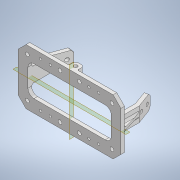
# Autodesk Inventor part: body_shell_1
Saved by Autodesk Inventor 2023 (Build 270158000, 158)
## iProperties
Created: 2021-02-28
Part Number: body_shell_1
Material: Generic
Document SubType Name: Modeling
Designer: Shuang Peng
Density: 1 g/cm^3
Appearance: Default
Author: Shuang Peng
Autodesk Inventor part; units mm, degrees
ref_plane "YZ Plane" through (0, 0, 0) normal (1, 0, 0) x (0, 1, 0)
ref_plane "XZ Plane" through (0, 0, 0) normal (0, 1, 0) x (-1, 0, 0)
ref_plane "XY Plane" through (0, 0, 0) normal (0, 0, 1) x (1, 0, 0)
sketch "Sketch1" plane through (0, 0, 0) normal (0, 0, 1) x (1, 0, 0)
  line L0 (0, -11) -> (-2, -13) projected
  line L1 (0, -4) -> (0, -11) projected
  line L2 (0, 0) -> (0, -4) projected
  line L3 (-15, 0) -> (0, 0) projected
  line L4 (-15, 0) -> (-15, -4) projected
  line L5 (-15, -4) -> (-15, -11) projected
  line L6 (-13, -13) -> (-15, -11) projected
  line L7 (-2, -13) -> (-13, -13) projected
  circle A0 centre (-3.5, -8.5) radius 1.6 projected
  circle A1 centre (-11.5, -8.5) radius 1.6 projected
  line L8 (25, -11) -> (27, -13) projected
  line L9 (27, -13) -> (38, -13) projected
  line L10 (38, -13) -> (40, -11) projected
  line L11 (40, -4) -> (40, -11) projected
  line L12 (40, 0) -> (40, -4) projected
  line L13 (40, 0) -> (25, 0) projected
  line L14 (25, 0) -> (25, -4) projected
  line L15 (25, -4) -> (25, -11) projected
  circle A2 centre (28.5, -8.5) radius 1.6 projected
  circle A3 centre (36.5, -8.5) radius 1.6 projected
  line L16 (0, 31) -> (-2, 33) projected
  line L17 (-2, 33) -> (-13, 33) projected
  line L18 (-13, 33) -> (-15, 31) projected
  line L19 (-15, 24) -> (-15, 31) projected
  line L20 (-15, 20) -> (-15, 24) projected
  line L21 (-15, 20) -> (0, 20) projected
  line L22 (0, 20) -> (0, 24) projected
  line L23 (0, 24) -> (0, 31) projected
  circle A4 centre (-3.5, 28.5) radius 1.6 projected
  circle A5 centre (-11.5, 28.5) radius 1.6 projected
  line L24 (25, 31) -> (27, 33) projected
  line L25 (25, 24) -> (25, 31) projected
  line L26 (25, 20) -> (25, 24) projected
  line L27 (40, 20) -> (25, 20) projected
  line L28 (40, 20) -> (40, 24) projected
  line L29 (40, 24) -> (40, 31) projected
  line L30 (38, 33) -> (40, 31) projected
  line L31 (27, 33) -> (38, 33) projected
  circle A6 centre (28.5, 28.5) radius 1.6 projected
  circle A7 centre (36.5, 28.5) radius 1.6 projected
  line L32 (-11.5, -8.5) -> (-3.5, -8.5)
  line L33 (28.5, -8.5) -> (36.5, -8.5)
  line L34 (-11.5, 28.5) -> (-3.5, 28.5)
  line L35 (28.5, 28.5) -> (36.5, 28.5)
  line L36 (28.5, -8.5) -> (-3.5, -8.5)
  line L37 (-3.5, 28.5) -> (28.5, 28.5)
  line L38 (-15, -14.5) -> (-15, -2.5)
  line L39 (-15, -2.5) -> (40, -2.5)
  line L40 (40, -2.5) -> (40, -14.5)
  line L41 (40, -14.5) -> (-15, -14.5)
  line L42 (-15, -14.5) -> (40, -2.5) construction
  line L43 (-15, -2.5) -> (40, -14.5) construction
  line L44 (-15, 22.5) -> (-15, 34.5)
  line L45 (-15, 34.5) -> (40, 34.5)
  line L46 (40, 34.5) -> (40, 22.5)
  line L47 (40, 22.5) -> (-15, 22.5)
  line L48 (-15, 22.5) -> (40, 34.5) construction
  line L49 (-15, 34.5) -> (40, 22.5) construction
  line L50 (-15, -14.5) -> (-25, -14.5)
  line L51 (-25, -14.5) -> (-25, 34.5)
  line L52 (-25, 34.5) -> (-15, 34.5)
  line L53 (-15, 34.5) -> (-15, -14.5)
  line L54 (40, -14.5) -> (50, -14.5)
  line L55 (50, -14.5) -> (50, 34.5)
  line L56 (50, 34.5) -> (40, 34.5)
  line L57 (40, 34.5) -> (40, -14.5)
  point P0 (12.5, -8.5)
  point P1 (12.5, 28.5)
  point P2 (-15, -2.5)
  dimension "d0" = 12
  dimension "d1" = 55
  dimension "d2" = 12
  dimension "d3" = 55
  dimension "d4" = 10
  dimension "d5" = 49
  dimension "d6" = 10
  dimension "d7" = 49
  constraints: 52 end point, 9 parallel, 7 perpendicular, 6 horizontal, 6 midpoint
  measures "d0" distance of L38.start L38.end
  measures "d1" distance of L38.end L39.end
  measures "d2" distance of L44.start L44.end
  measures "d3" distance of L44.end L45.end
  measures "d4" distance of L51.end L52.end
  measures "d5" distance of L50.end L51.end
  measures "d6" distance of L55.end L56.end
  measures "d7" distance of L54.end L55.end
extrude "Extrusion1" add sketch "Sketch1" along normal blind 3 contours L1 L36 L15 L8 L9 L10 L40 L41 L38 L6 L7 L0 | L0 L7 L6 L5 L4 L39 L2 L1 | L1 L2 L39 L14 L15 L36 | L15 L14 L39 L12 L11 L10 L9 L8 | L38 L50 L51 L52 L44 L19 L20 L53 L4 L5 | L40 L11 L12 L57 L28 L29 L46 L56 L55 L54 | L45 L46 L30 L31 L24 L25 L37 L23 L16 L17 L18 L44 | L20 L19 L18 L17 L16 L23 L22 L47 | L22 L23 L37 L25 L26 L47 | L47 L26 L25 L24 L31 L30 L29 L28
sketch "Sketch2" plane through (0, 0, 3) normal (0, 0, 1) x (1, 0, 0)
  line L0 (50, -14.5) -> (50, 34.5) projected
  line L1 (50, 34.5) -> (-25, 34.5) projected
  line L2 (-25, 34.5) -> (-25, -14.5) projected
  line L3 (-25, -14.5) -> (50, -14.5) projected
  circle A0 centre (36.5, -8.5) radius 1.6 projected
  circle A1 centre (28.5, -8.5) radius 1.6 projected
  circle A2 centre (-11.5, 28.5) radius 1.6 projected
  circle A3 centre (-3.5, 28.5) radius 1.6 projected
  circle A4 centre (36.5, 28.5) radius 1.6 projected
  circle A5 centre (28.5, 28.5) radius 1.6 projected
  circle A6 centre (-3.5, -8.5) radius 1.6 projected
  circle A7 centre (-11.5, -8.5) radius 1.6 projected
  line L4 (-15, -2.5) -> (-15, 22.5) projected
  line L5 (-15, 22.5) -> (40, 22.5) projected
  line L6 (40, 22.5) -> (40, -2.5) projected
  line L7 (40, -2.5) -> (-15, -2.5) projected
  circle A8 centre (36.5, 28.5) radius 1.6 projected
  circle A9 centre (36.5, 28.5) radius 1
  circle A10 centre (28.5, 28.5) radius 1.6 projected
  circle A11 centre (28.5, 28.5) radius 1
  circle A12 centre (-3.5, 28.5) radius 1
  circle A13 centre (-11.5, 28.5) radius 1.6 projected
  circle A14 centre (-11.5, 28.5) radius 1
  circle A15 centre (-3.5, -8.5) radius 1.6 projected
  circle A16 centre (-3.5, -8.5) radius 1
  circle A17 centre (-11.5, -8.5) radius 1
  circle A18 centre (28.5, -8.5) radius 1.6 projected
  circle A19 centre (28.5, -8.5) radius 1
  circle A20 centre (36.5, -8.5) radius 1
  point P0 (0, 0)
  dimension "d10" = 2
  dimension "d11" = 2
  dimension "d12" = 2
  dimension "d13" = 2
  dimension "d14" = 2
  dimension "d15" = 2
  dimension "d16" = 2
  dimension "d17" = 2
  constraints: 8 centre point, 8 coincident
  measures "d10" diameter of A9
  measures "d11" diameter of A11
  measures "d12" diameter of A12
  measures "d13" diameter of A14
  measures "d14" diameter of A16
  measures "d15" diameter of A17
  measures "d16" diameter of A19
  measures "d17" diameter of A20
extrude "Extrusion2" add sketch "Sketch2" against normal up to surface (3 mm away) contours A0 | A1 | A2 | A3 | A4 | A5 | A6 | A7
thicken "Thicken1" operation add thickness 5 both sides no extend neighbours yes toward (-1, 0, 0) faces at (-25, 18.1667, 1)
thicken "Thicken2" operation add thickness 7 both sides no extend neighbours yes toward (-1, 0, 0) faces at (-15, 5.8333, 1)
thicken "Thicken3" operation add thickness 5 both sides no extend neighbours yes toward (1, 0, 0) faces at (50, 1.8333, 1)
thicken "Thicken4" operation add thickness 7 both sides no extend neighbours yes toward (1, 0, 0) faces at (40, 14.1667, 1)
ref_plane "Work Plane1" through (12.5, -14.5, 0) normal (-1, 0, 0) x (0, 0, 1)
sketch "Sketch3" plane through (-30, -14.5, 0) normal (0, -1, 0) x (1, 0, 0)
  point P0 (30, 0)
ref_plane "Work Plane2" through (-30, 10, 0) normal (0, -1, 0) x (1, 0, 0)
sketch "Sketch4" plane through (-30, 10, 0) normal (0, -1, 0) x (1, 0, 0)
  line L0 (12.8994, -48) -> (19, -48) projected
  line L1 (19, -45) -> (19, -48) projected
  line L2 (15, -45) -> (19, -45) projected
  line L3 (15, -45) -> (4.7394, -16.8092) projected
  line L4 (4.7394, -16.8092) -> (1.5469, -16.8092) projected
  line L5 (1.5469, -16.8092) -> (12.8994, -48) projected
  line L6 (26, -45) -> (9.8697, -30.9046) projected
  line L7 (9.8697, -30.9046) -> (12.8272, -30.2589)
  line L8 (0, 0) -> (85, 0) projected
  line L9 (85, 0) -> (85, 3) projected
  line L10 (0, 3) -> (85, 3) projected
  line L11 (0, 0) -> (0, 3) projected
  line L12 (4.7394, -16.8092) -> (4.7394, 0)
  line L13 (85, 0) -> (0, 0) projected
  line L14 (12.8272, -30.2589) -> (7.7394, -16.2802)
  line L15 (7.7394, -16.2802) -> (7.7394, 0)
  point P0 (30, 0)
  dimension "d28" = 3
  dimension "d29" = 3
  constraints: 8 end point, 2 perpendicular, 2 point on line, 1 parallel
  measures "d28" distance between parallel lines of L12 L15
  measures "d29" distance between parallel lines of L3 L14
extrude "Extrusion3" add sketch "Sketch4" along normal mid plane 12 contours L12 L8 L15 L14 L7 L3
sketch "Sketch5" plane through (-30, 10, 0) normal (0, -1, 0) x (1, 0, 0)
  line L0 (7.7394, 0) -> (4.7394, 0) projected
  line L1 (7.7394, 0) -> (7.7394, -16.2802) projected
  line L2 (7.7394, -16.2802) -> (12.8272, -30.2589) projected
  line L3 (12.8272, -30.2589) -> (9.8697, -30.9046) projected
  line L4 (9.8697, -30.9046) -> (4.7394, -16.8092) projected
  line L5 (4.7394, -16.8092) -> (4.7394, 0) projected
  line L6 (85, 0) -> (0, 0) projected
  line L7 (0, 0) -> (0, 3) projected
  line L8 (85, 3) -> (0, 3) projected
  line L9 (85, 0) -> (85, 3) projected
  line L10 (0, 0) -> (4.7394, -16.8092)
  point P0 (30, 0)
  constraints: 2 end point
extrude "Extrusion4" add sketch "Sketch5" along normal mid plane 2 contours L5 L10 L6
mirror "Mirror1" about plane through (12.5, -14.5, 0) normal (-1, 0, 0) of "Extrusion3", "Extrusion4"
sketch "Sketch6" plane through (-30, 16, 0) normal (0, 1, 0) x (1, 0, 0)
  line L0 (7.7394, 0) -> (4.7394, 0) projected
  line L1 (7.7394, 0) -> (7.7394, 16.2802) projected
  line L2 (7.7394, 16.2802) -> (12.8272, 30.2589) projected
  line L3 (12.8272, 30.2589) -> (9.8697, 30.9046) projected
  line L4 (9.8697, 30.9046) -> (4.7394, 16.8092) projected
  line L5 (4.7394, 16.8092) -> (4.7394, 0) projected
  line L6 (8, 0) -> (8, -3) projected
  line L7 (80.2606, 0) -> (85, 0) projected
  line L8 (0, 0) -> (85, 0) projected
  line L9 (0, 0) -> (4.7394, 0) projected
  line L10 (4.7394, 0) -> (7.7394, 0) projected
  line L11 (7.7394, 0) -> (4.7394, 0) projected
  line L12 (4.7394, 0) -> (0, 0) projected
  line L13 (85, 0) -> (0, 0) projected
  line L14 (85, 0) -> (80.2606, 0) projected
  line L15 (80.2606, 0) -> (77.2606, 0) projected
  line L16 (77.2606, 0) -> (80.2606, 0) projected
  line L17 (77, 0) -> (8, 0) projected
  line L18 (8, 0) -> (77, 0) projected
  line L19 (57.5, 0) -> (59.5, 0) projected
  line L20 (17.5, 0) -> (19.5, 0) projected
  line L21 (57.5, 0) -> (59.5, 0) projected
  line L22 (25.5, 0) -> (27.5, 0) projected
  line L23 (65.5, 0) -> (67.5, 0) projected
  line L24 (25.5, 0) -> (27.5, 0) projected
  line L25 (65.5, 0) -> (67.5, 0) projected
  line L26 (17.5, 0) -> (19.5, 0) projected
  line L27 (8, 0) -> (8, 16.9962)
  line L28 (7.7394, 0) -> (7.7394, 16.2802) projected
  point P0 (30, 0)
  constraints: 2 end point, 1 parallel, 1 point on line
extrude "Extrusion5" add sketch "Sketch6" against normal up to surface (12 mm away) contours L1 L2 L27 L8
mirror "Mirror2" about plane through (12.5, -14.5, 0) normal (-1, 0, 0) of "Extrusion5"
sketch "Sketch7" plane through (45.1303, 4, -30.9046) normal (0.9396926, 0, -0.3420201) x (-0.3420201, 0, -0.9396926)
  line L0 (0, 12) -> (0, 0) projected
  line L1 (0, 12) -> (-15, 12) projected
  line L2 (-15, 12) -> (-15, 7) projected
  line L3 (-15, 7) -> (-15, 5) projected
  line L4 (-15, 5) -> (-15, 0) projected
  line L5 (-15, 0) -> (0, 0) projected
  line L6 (0, 6) -> (-4, 6)
  line L7 (-6.1638, 30.5) -> (-6.1638, -18.5) projected
  line L8 (-4, 6) -> (-12, 6)
  circle A0 centre (-12, 6) radius 1.55
  circle A1 centre (-4, 6) radius 1.55
  point P0 (-13.6054, -4)
  dimension "d36" = 4
  dimension "d37" = 8
  dimension "d38" = 3.1
  dimension "d39" = 3.1
  constraints: 4 end point, 2 centre point, 2 coincident, 1 midpoint, 1 perpendicular, 1 point on line
  measures "d36" distance of L6.start L6.end
  measures "d37" distance of L6.end L8.end
  measures "d38" diameter of A0
  measures "d39" diameter of A1
extrude "Extrusion6" cut sketch "Sketch7" against normal up to surface (3 mm away) contours A1 L8 L6 | L6 L8 A1 | A0
mirror "Mirror3" about plane through (12.5, -14.5, 0) normal (-1, 0, 0) of "Extrusion6"
sketch "Sketch8" plane through (0, 0, 3) normal (0, 0, 1) x (1, 0, 0)
  circle A0 centre (-11.5, 28.5) radius 1 projected
  circle A1 centre (36.5, 28.5) radius 1 projected
  circle A2 centre (-3.5, -8.5) radius 1 projected
  circle A3 centre (36.5, -8.5) radius 1 projected
  circle A4 centre (-3.5, 28.5) radius 1 projected
  circle A5 centre (28.5, 28.5) radius 1 projected
  circle A6 centre (-11.5, -8.5) radius 1 projected
  circle A7 centre (28.5, -8.5) radius 1 projected
  line L0 (55, -14.5) -> (55, 34.5) projected
  line L1 (55, 34.5) -> (-30, 34.5) projected
  line L2 (-30, 34.5) -> (-30, -14.5) projected
  line L3 (-30, -14.5) -> (55, -14.5) projected
  line L4 (-22, -2.5) -> (-22, 22.5) projected
  line L5 (-22, 22.5) -> (47, 22.5) projected
  line L6 (47, 22.5) -> (47, -2.5) projected
  line L7 (47, -2.5) -> (-22, -2.5) projected
  line L8 (28.5, 28.5) -> (-3.5, 28.5)
  line L9 (12.5, 28.5) -> (4.5, 28.5)
  line L10 (12.5, 28.5) -> (20.5, 28.5)
  circle A8 centre (20.5, 28.5) radius 1.55
  circle A9 centre (4.5, 28.5) radius 1.55
  point P0 (0, 0)
  dimension "d45" = 8
  dimension "d46" = 8
  dimension "d47" = 3.1
  dimension "d48" = 3.1
  constraints: 6 end point, 2 centre point, 2 coincident, 2 point on line, 1 horizontal, 1 midpoint
  measures "d45" distance of L9.start L9.end
  measures "d46" distance of L9.start L10.end
  measures "d47" diameter of A8
  measures "d48" diameter of A9
extrude "Extrusion7" cut sketch "Sketch8" against normal blind 10 contours A8 L8 | L8 A8 | A9 L8 | L8 A9
mirror "Mirror4" about plane through (-30, 10, 0) normal (0, -1, 0) of "Extrusion7"
sketch "Sketch9" plane through (-30, 34.5, 3) normal (0, 1, 0) x (1, 0, 0)
  line L0 (85, 3) -> (0, 3) projected
  line L1 (0, 3) -> (0, 0) projected
  line L2 (85, 0) -> (0, 0) projected
  line L3 (85, 3) -> (85, 0) projected
  line L4 (42.5, 3) -> (42.5, 5)
  line L5 (46, 1.5) -> (39, 1.5)
  line L6 (39, 1.5) -> (39, 8.5)
  line L7 (39, 8.5) -> (46, 8.5)
  line L8 (46, 8.5) -> (46, 1.5)
  line L9 (46, 1.5) -> (39, 8.5) construction
  line L10 (39, 1.5) -> (46, 8.5) construction
  circle A0 centre (42.5, 5) radius 1.55
  point P0 (30, 3)
  point P1 (46, 3)
  point P2 (39, 3)
  dimension "d51" = 2
  dimension "d52" = 7
  dimension "d53" = 7
  dimension "d54" = 3.1
  constraints: 14 end point, 3 midpoint, 2 parallel, 2 perpendicular, 1 centre point, 1 coincident, 1 vertical
  measures "d51" distance of L4.start L4.end
  measures "d52" distance of L5.start L5.end
  measures "d53" distance of L5.end L6.end
  measures "d54" diameter of A0
extrude "Extrusion8" add sketch "Sketch9" against normal blind 5 contours L0 L6 L7 L8
mirror "Mirror5" about plane through (-30, 10, 0) normal (0, -1, 0) of "Extrusion8"
chamfer "Chamfer2" distance 1.5 angle 45 4 edges at (9, 32, -5.5) (16, 32, -5.5) (16, -12, -5.5) (9, -12, -5.5)
fillet "Fillet1" radius 2 2 edges at (12.5, -9.5, 0) (12.5, 29.5, 0)
fillet "Fillet2" radius 5 4 edges at (-22, 22.5, 1.5) (-22, -2.5, 1.5) (47, -2.5, 1.5) (47, 22.5, 1.5)
chamfer "Chamfer3" distance 8 angle 45 4 edges at (-30, 34.5, 1.5) (-30, -14.5, 1.5) (55, -14.5, 1.5) (55, 34.5, 1.5)
sketch "Sketch10" plane through (0, 0, 3) normal (0, 0, 1) x (1, 0, 0)
  line L0 (47, 34.5) -> (55, 26.5) projected
  line L1 (47, 34.5) -> (-22, 34.5) projected
  line L2 (-30, 26.5) -> (-22, 34.5) projected
  line L3 (-30, 26.5) -> (-30, -6.5) projected
  line L4 (-22, -14.5) -> (-30, -6.5) projected
  line L5 (-22, -14.5) -> (47, -14.5) projected
  line L6 (55, -6.5) -> (47, -14.5) projected
  line L7 (55, -6.5) -> (55, 26.5) projected
  circle A0 centre (4.5, -8.5) radius 1.55 projected
  circle A1 centre (20.5, -8.5) radius 1.55 projected
  circle A2 centre (4.5, 28.5) radius 1.55 projected
  circle A3 centre (20.5, 28.5) radius 1.55 projected
  circle A4 centre (-11.5, 28.5) radius 1 projected
  circle A5 centre (36.5, 28.5) radius 1 projected
  circle A6 centre (-3.5, -8.5) radius 1 projected
  circle A7 centre (36.5, -8.5) radius 1 projected
  circle A8 centre (-3.5, 28.5) radius 1 projected
  circle A9 centre (28.5, 28.5) radius 1 projected
  circle A10 centre (-11.5, -8.5) radius 1 projected
  circle A11 centre (28.5, -8.5) radius 1 projected
  line L8 (-22, 2.5) -> (-22, 17.5) projected
  arc A12 (-17, 22.5) -> (-22, 17.5) centre (-17, 17.5) ccw projected
  line L9 (-17, 22.5) -> (42, 22.5) projected
  arc A13 (47, 17.5) -> (42, 22.5) centre (42, 17.5) ccw projected
  line L10 (47, 17.5) -> (47, 2.5) projected
  arc A14 (42, -2.5) -> (47, 2.5) centre (42, 2.5) ccw projected
  line L11 (42, -2.5) -> (-17, -2.5) projected
  arc A15 (-22, 2.5) -> (-17, -2.5) centre (-17, 2.5) ccw projected
  line L12 (-17, 17.5) -> (42, 2.5)
  line L13 (-17, 2.5) -> (42, 17.5)
  line L14 (-22.5, 26.5) -> (-22.5, -6.5)
  line L15 (-22.5, -6.5) -> (47.5, -6.5)
  line L16 (47.5, -6.5) -> (47.5, 26.5)
  line L17 (47.5, 26.5) -> (-22.5, 26.5)
  line L18 (-22.5, 26.5) -> (47.5, -6.5) construction
  line L19 (-22.5, -6.5) -> (47.5, 26.5) construction
  point P0 (0, 0)
  point P1 (12.5, 10)
  dimension "d65" = 33
  dimension "d66" = 70
  constraints: 16 end point, 3 midpoint, 2 parallel, 1 perpendicular, 1 vertical
  measures "d65" distance of L14.start L14.end
  measures "d66" distance of L15.end L14.end
hole "Hole1" at (47.5, 26.5, 3) at (47.5, -6.5, 3) at (-22.5, -6.5, 3) at (-22.5, 26.5, 3) direction (0, 0, -1) diameter 3.1 depth 20
fillet "Fillet3" radius 2 8 edges at (-23.6303, 4, 0) (-23.6303, 16, 0) (48.6303, 16, 0) (48.6303, 4, 0) (50.2606, 6.5, 0) (50.2606, 13.5, 0) (-25.2606, 6.5, 0) (-25.2606, 13.5, 0)
fillet "Fillet4" radius 1.5 12 edges at (-28.6303, 9, 0) (-25.2606, 9, -9.4046) (-25.8464, 9, -0.5858) (-25.8464, 11, -0.5858) (-28.6303, 11, 0) (-25.2606, 11, -9.4046) (53.6303, 11, 0) (50.2606, 11, -9.4046) (50.8464, 11, -0.5858) (50.2606, 9, -9.4046) (53.6303, 9, 0) (50.8464, 9, -0.5858)
chamfer "Chamfer4" distance 2 angle 45 4 edges at (43.6515, 4, -30.5818) (43.6515, 16, -30.5818) (-18.6515, 4, -30.5818) (-18.6515, 16, -30.5818)
thicken "Thicken5" operation add thickness 1.5 both sides no extend neighbours yes toward (0, 1, 0) faces at (11.3333, -14.5, 2)
thicken "Thicken6" operation add thickness 1.5 both sides no extend neighbours yes toward (0, 1, 0) faces at (12.5623, -9.5, -4.8462)
thicken "Thicken7" operation add thickness 1.5 both sides no extend neighbours yes toward (0, -1, 0) faces at (11.3333, 34.5, 2)
thicken "Thicken8" operation add thickness 1.5 both sides no extend neighbours yes toward (0, -1, 0) faces at (12.5623, 29.5, -4.8462)
fillet "Fillet5" radius 1 4 edges at (16, 29.5, 0) (9, 29.5, 0) (9, -9.5, 0) (16, -9.5, 0)
sketch "Sketch11" plane through (0, 0, 3) normal (0, 0, 1) x (1, 0, 0)
  circle A0 centre (-22.5, -6.5) radius 1.55 projected
  circle A1 centre (47.5, 26.5) radius 1.55 projected
  circle A2 centre (47.5, -6.5) radius 1.55 projected
  circle A3 centre (-22.5, 26.5) radius 1.55 projected
  line L0 (48.5, 33) -> (55, 26.5) projected
  line L1 (48.5, 33) -> (-23.5, 33) projected
  line L2 (-30, 26.5) -> (-23.5, 33) projected
  line L3 (-30, 26.5) -> (-30, -6.5) projected
  line L4 (-23.5, -13) -> (-30, -6.5) projected
  line L5 (-23.5, -13) -> (48.5, -13) projected
  line L6 (55, -6.5) -> (48.5, -13) projected
  line L7 (55, -6.5) -> (55, 26.5) projected
  circle A4 centre (4.5, -8.5) radius 1.55 projected
  circle A5 centre (20.5, -8.5) radius 1.55 projected
  circle A6 centre (4.5, 28.5) radius 1.55 projected
  circle A7 centre (20.5, 28.5) radius 1.55 projected
  circle A8 centre (-11.5, 28.5) radius 1 projected
  circle A9 centre (36.5, 28.5) radius 1 projected
  circle A10 centre (-3.5, -8.5) radius 1 projected
  circle A11 centre (36.5, -8.5) radius 1 projected
  circle A12 centre (-3.5, 28.5) radius 1 projected
  circle A13 centre (28.5, 28.5) radius 1 projected
  circle A14 centre (-11.5, -8.5) radius 1 projected
  circle A15 centre (28.5, -8.5) radius 1 projected
  line L8 (-22, 2.5) -> (-22, 17.5) projected
  arc A16 (-17, 22.5) -> (-22, 17.5) centre (-17, 17.5) ccw projected
  line L9 (-17, 22.5) -> (42, 22.5) projected
  arc A17 (47, 17.5) -> (42, 22.5) centre (42, 17.5) ccw projected
  line L10 (47, 17.5) -> (47, 2.5) projected
  arc A18 (42, -2.5) -> (47, 2.5) centre (42, 2.5) ccw projected
  line L11 (42, -2.5) -> (-17, -2.5) projected
  arc A19 (-22, 2.5) -> (-17, -2.5) centre (-17, 2.5) ccw projected
  line L12 (-17, 22.5) -> (42, 22.5) projected
  line L13 (12.5, 22.5) -> (12.5, -2.5)
  line L14 (15.5, -2.5) -> (9.5, -2.5)
  line L15 (9.5, -2.5) -> (9.5, 22.5)
  line L16 (9.5, 22.5) -> (15.5, 22.5)
  line L17 (15.5, 22.5) -> (15.5, -2.5)
  line L18 (15.5, -2.5) -> (9.5, 22.5) construction
  line L19 (9.5, -2.5) -> (15.5, 22.5) construction
  point P0 (0, 0)
  point P1 (12.5, 10)
  point P2 (15.5, -2.5)
  point P3 (15.5, 22.5)
  point P4 (9.5, 22.5)
  point P5 (9.5, -2.5)
  dimension "d88" = 6
  dimension "d89" = 25
  constraints: 14 end point, 5 midpoint, 2 parallel, 2 perpendicular
  measures "d88" distance of L14.start L14.end
  measures "d89" distance of L14.end L15.end
extrude "Extrusion9" add sketch "Sketch11" against normal up to surface (3 mm away) contours L15 L9 L13 L11 | L13 L9 L17 L11
fillet "Fillet6" radius 3 4 edges at (15.5, -2.5, 1.5) (9.5, -2.5, 1.5) (9.5, 22.5, 1.5) (15.5, 22.5, 1.5)
body "Solid1"
